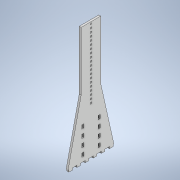
# Autodesk Inventor part: mdf_vertical_r1
Saved by Autodesk Inventor 2021.2 (Build 252289000, 289)
## iProperties
Created: 2021-03-24
Part Number: mdf_vertical_r1
Material: Generic
Document SubType Name: Modeling
Designer: yxion
Density: 1 g/cm^3
Appearance: Default
Author: yxion
Autodesk Inventor part; units mm, degrees
ref_plane "YZ Plane" through (0, 0, 0) normal (1, 0, 0) x (0, 1, 0)
ref_plane "XZ Plane" through (0, 0, 0) normal (0, 1, 0) x (-1, 0, 0)
ref_plane "XY Plane" through (0, 0, 0) normal (0, 0, 1) x (1, 0, 0)
sketch "Sketch1" plane through (0, 0, 0) normal (1, 0, 0) x (0, 1, 0)
  line L0 (0, 0) -> (0, -152.4) construction
  line L1 (390, -43.7) -> (0, -43.7) construction
  line L2 (0, -43.7) -> (0, -108.7) construction
  line L3 (0, -108.7) -> (390, -108.7) construction
  line L4 (390, -108.7) -> (390, -43.7) construction
  line L5 (0, 0) -> (0, -152.4)
  line L6 (0, 0) -> (195, -43.7)
  line L7 (0, -152.4) -> (195, -108.7)
  line L8 (195, -43.7) -> (390, -43.7)
  line L9 (390, -43.7) -> (390, -108.7)
  line L10 (390, -108.7) -> (195, -108.7)
  circle A0 centre (384, -76.2) radius 2.875
  line L11 (390, -66.2) -> (366, -66.2)
  line L12 (366, -86.2) -> (390, -86.2)
  line L13 (390, -86.2) -> (390, -66.2)
  circle A1 centre (372, -76.2) radius 2.875
  line L14 (0, -2.7) -> (-6.4, -2.7)
  line L15 (-6.4, -2.7) -> (-6.4, -14.7)
  line L16 (-6.4, -14.7) -> (0, -14.7)
  line L17 (0, -14.7) -> (0, -2.7)
  line L18 (-6.4, -29.7) -> (-6.4, -41.7)
  line L19 (-6.4, -41.7) -> (0, -41.7)
  line L20 (0, -29.7) -> (-6.4, -29.7)
  line L21 (-6.4, -56.7) -> (-6.4, -68.7)
  line L22 (-6.4, -68.7) -> (0, -68.7)
  line L23 (0, -56.7) -> (-6.4, -56.7)
  line L24 (-6.4, -83.7) -> (-6.4, -95.7)
  line L25 (-6.4, -95.7) -> (0, -95.7)
  line L26 (0, -83.7) -> (-6.4, -83.7)
  line L27 (-6.4, -110.7) -> (-6.4, -122.7)
  line L28 (-6.4, -122.7) -> (0, -122.7)
  line L29 (0, -110.7) -> (-6.4, -110.7)
  line L30 (-6.4, -137.7) -> (-6.4, -149.7)
  line L31 (-6.4, -149.7) -> (0, -149.7)
  line L32 (0, -137.7) -> (-6.4, -137.7)
  line L33 (27, -46) -> (15, -46)
  line L34 (15, -46) -> (15, -52.4)
  line L35 (15, -52.4) -> (27, -52.4)
  line L36 (27, -52.4) -> (27, -46)
  line L37 (27, -49.2) -> (15, -49.2) construction
  line L38 (42, -52.4) -> (54, -52.4)
  line L39 (54, -46) -> (42, -46)
  line L40 (42, -46) -> (42, -52.4)
  line L41 (54, -52.4) -> (54, -46)
  line L42 (69, -52.4) -> (81, -52.4)
  line L43 (81, -46) -> (69, -46)
  line L44 (69, -46) -> (69, -52.4)
  line L45 (81, -52.4) -> (81, -46)
  line L46 (96, -52.4) -> (108, -52.4)
  line L47 (108, -46) -> (96, -46)
  line L48 (96, -46) -> (96, -52.4)
  line L49 (108, -52.4) -> (108, -46)
  line L50 (96, -106.4) -> (108, -106.4)
  line L51 (108, -100) -> (96, -100)
  line L52 (96, -100) -> (96, -106.4)
  line L53 (108, -106.4) -> (108, -100)
  line L54 (69, -106.4) -> (81, -106.4)
  line L55 (69, -100) -> (69, -106.4)
  line L56 (81, -100) -> (69, -100)
  line L57 (81, -106.4) -> (81, -100)
  line L58 (42, -106.4) -> (54, -106.4)
  line L59 (54, -100) -> (42, -100)
  line L60 (54, -106.4) -> (54, -100)
  line L61 (42, -100) -> (42, -106.4)
  line L62 (15, -106.4) -> (27, -106.4)
  line L63 (15, -100) -> (15, -106.4)
  line L64 (27, -100) -> (15, -100)
  line L65 (27, -106.4) -> (27, -100)
  line L66 (366, -66.2) -> (366, -86.2)
  circle A2 centre (360, -76.2) radius 2.875
  circle A3 centre (348, -76.2) radius 2.875
  line L67 (366, -66.2) -> (342, -66.2)
  line L68 (342, -86.2) -> (366, -86.2)
  line L69 (342, -66.2) -> (342, -86.2)
  circle A4 centre (336, -76.2) radius 2.875
  circle A5 centre (324, -76.2) radius 2.875
  line L70 (342, -66.2) -> (318, -66.2)
  line L71 (318, -86.2) -> (342, -86.2)
  line L72 (318, -66.2) -> (318, -86.2)
  circle A6 centre (312, -76.2) radius 2.875
  circle A7 centre (300, -76.2) radius 2.875
  line L73 (318, -66.2) -> (294, -66.2)
  line L74 (294, -86.2) -> (318, -86.2)
  line L75 (294, -66.2) -> (294, -86.2)
  circle A8 centre (288, -76.2) radius 2.875
  circle A9 centre (276, -76.2) radius 2.875
  line L76 (294, -66.2) -> (270, -66.2)
  line L77 (270, -86.2) -> (294, -86.2)
  line L78 (270, -66.2) -> (270, -86.2)
  circle A10 centre (264, -76.2) radius 2.875
  circle A11 centre (252, -76.2) radius 2.875
  line L79 (270, -66.2) -> (246, -66.2)
  line L80 (246, -86.2) -> (270, -86.2)
  line L81 (246, -66.2) -> (246, -86.2)
  circle A12 centre (240, -76.2) radius 2.875
  circle A13 centre (228, -76.2) radius 2.875
  line L82 (246, -66.2) -> (222, -66.2)
  line L83 (222, -86.2) -> (246, -86.2)
  line L84 (222, -66.2) -> (222, -86.2)
  circle A14 centre (216, -76.2) radius 2.875
  circle A15 centre (204, -76.2) radius 2.875
  line L85 (222, -66.2) -> (198, -66.2)
  line L86 (198, -86.2) -> (222, -86.2)
  line L87 (198, -66.2) -> (198, -86.2)
  circle A16 centre (192, -76.2) radius 2.875
  circle A17 centre (180, -76.2) radius 2.875
  line L88 (198, -66.2) -> (174, -66.2)
  line L89 (174, -86.2) -> (198, -86.2)
  line L90 (174, -66.2) -> (174, -86.2)
  circle A18 centre (168, -76.2) radius 2.875
  circle A19 centre (156, -76.2) radius 2.875
  line L91 (174, -66.2) -> (150, -66.2)
  line L92 (150, -86.2) -> (174, -86.2)
  line L93 (150, -66.2) -> (150, -86.2)
  point P0 (390, -86.2)
  point P1 (390, -66.2)
  point P2 (0, -8.7)
  point P3 (0, -149.7)
  point P4 (0, -122.7)
  point P5 (0, -95.7)
  point P6 (0, -68.7)
  point P7 (0, -41.7)
  point P8 (117.4088, -76.2)
  point P9 (42, -49.2)
  point P10 (54, -49.2)
  point P11 (69, -49.2)
  point P12 (81, -49.2)
  point P13 (96, -49.2)
  point P14 (108, -49.2)
  point P15 (108, -103.2)
  point P16 (96, -103.2)
  point P17 (69, -103.2)
  point P18 (81, -103.2)
  point P19 (54, -103.2)
  point P20 (42, -103.2)
  point P21 (15, -103.2)
  point P22 (27, -103.2)
  dimension "d0" = 152.4
  dimension "d1" = 65
  dimension "d2" = 390
  dimension "d4" = 5.75
  dimension "d5" = 20
  dimension "d8" = 5.75
  dimension "d11" = 0
  dimension "d21" = 12
  dimension "d22" = 6.4
  dimension "d23" = 2.7
  dimension "d26" = 27
  dimension "d39" = 12
  dimension "d40" = 6.4
  dimension "d41" = 46
  dimension "d42" = 15
  dimension "d45" = 27
  dimension "d52" = 54
  dimension "d57" = 12
  dimension "d58" = 6
  dimension "d59" = 6
  dimension "d62" = 24
  constraints: 188 end point, 20 centre point, 8 collinear, 7 parallel, 6 horizontal, 5 midpoint, 5 vertical, 3 perpendicular, 1 coincident, 1 point on line, 200 other
  measures "d0" distance of L0.start L0.end
  measures "d1" distance of L3.end L1.start
  measures "d2" distance between parallel lines of L2 L4
  measures "d4" diameter of A0
  measures "d5" distance of L12.end L11.start
  measures "d8" diameter of A1
  measures "d11" distance between parallel lines of L13 L4
  measures "d21" distance of L14.end L15.end
  measures "d22" distance of L15.end L16.end
  measures "d23" distance from line of L14 point (0, 0)
  measures "d26" distance of L14.end L18.start
  measures "d39" distance of L34.end L35.end
  measures "d40" distance of L35.end L33.start
  measures "d41" distance from line of point (0, 0) L33
  measures "d42" distance between parallel lines of L2 L34
  measures "d45" distance of L34.end L38.start
  measures "d52" distance of L46.start L50.start
  measures "d57" distance of A1.centre A0.centre
  measures "d58" distance from line of L13 A0.centre
  measures "d59" distance from line of L66 A1.centre
  measures "d62" distance of A0.centre A2.centre
extrude "Extrusion1" add sketch "Sketch1" along normal blind 6.4
body "Solid1"
